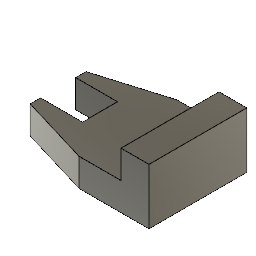
new (Autodesk Fusion 360 design; units mm, degrees)
Autodesk Fusion 360 part; units mm, degrees
sketch "Sketch1" plane through (0, 0, 0) normal (0, 0, 1) x (1, 0, 0)
  line L0 (97.7238, 100.1373) -> (197.7238, 100.1373)
  line L1 (197.7238, 100.1373) -> (197.7238, 30.1373)
  line L2 (197.7238, 30.1373) -> (97.7238, 30.1373)
  line L3 (97.7238, 30.1373) -> (97.7238, 100.1373)
  dimension "d1" = 70
  dimension "d2" = 100
  constraint horizontal L0
  constraint vertical L1
  constraint horizontal L2
  constraint vertical L3
  measures "d1" distance of L0.start L2.end
  measures "d2" distance of L1.end L2.end
extrude "Extrude1" add sketch "Sketch1" along normal blind 20
sketch "Sketch2" plane through (0, 0, 20) normal (0, 0, 1) x (-1, 0, 0)
  line L0 (-97.7238, -30.1373) -> (-197.7238, -30.1373)
  line L1 (-197.7238, -30.1373) -> (-197.7238, -100.1373)
  line L2 (-197.7238, -100.1373) -> (-97.7238, -100.1373)
  line L3 (-97.7238, -100.1373) -> (-97.7238, -30.1373)
  line L4 (-97.7238, -77.6373) -> (-127.7238, -77.6373)
  line L5 (-127.7238, -77.6373) -> (-127.7238, -52.6373)
  line L6 (-127.7238, -52.6373) -> (-97.7238, -52.6373)
  dimension "d5" = 22.5
  dimension "d6" = 22.5
  dimension "d7" = 25
  dimension "d8" = 30
  dimension "d9" = 25
  constraint coincident L3 L6.end
  constraint perpendicular L4 L5
  measures "d5" distance of L2.end L4.start
  measures "d6" distance of L0.start L6.end
  measures "d7" distance of L4.start L6.end
  measures "d8" distance of L4.start L4.end
  measures "d9" distance of L4.end L5.end
extrude "Extrude2" cut sketch "Sketch2" against normal blind 27.453 contours L3 L4 L5 L6
sketch "Sketch3" plane through (0, 0, 20) normal (0, 0, 1) x (-1, 0, 0)
  line L0 (-127.7238, -52.6373) -> (-97.7238, -52.6373)
  line L1 (-97.7238, -52.6373) -> (-97.7238, -30.1373)
  line L2 (-97.7238, -30.1373) -> (-197.7238, -30.1373)
  line L3 (-197.7238, -30.1373) -> (-197.7238, -100.1373)
  line L4 (-197.7238, -100.1373) -> (-97.7238, -100.1373)
  line L5 (-97.7238, -100.1373) -> (-97.7238, -77.6373)
  line L6 (-97.7238, -77.6373) -> (-127.7238, -77.6373)
  line L7 (-127.7238, -77.6373) -> (-127.7238, -52.6373)
  line L8 (-97.7238, -52.6373) -> (-97.7238, -45.1373)
  line L9 (-97.7238, -77.6373) -> (-97.7238, -85.1373)
  line L10 (-147.7238, -30.1373) -> (-147.7238, -100.1373)
  line L11 (-97.7238, -85.1373) -> (-147.7238, -100.1373)
  line L12 (-97.7238, -45.1373) -> (-147.7238, -30.1373)
  dimension "d12" = 7.5
  dimension "d13" = 7.5
  constraint coincident L0.end L1.start
  constraint perpendicular L0 L8
  constraint coincident L5.end L6.start
  constraint coincident L5 L9.end
  constraint midpoint L4 L10.end
  constraint midpoint L2 L10.start
  measures "d12" distance of L0.end L8.end
  measures "d13" distance of L5.end L9.end
extrude "Extrude3" cut sketch "Sketch3" against normal blind 62.472 contours L1 L2 L12
extrude "Extrude4" cut sketch "Sketch3" against normal blind 73.462 contours L4 L5 L11
sketch "Sketch4" plane through (0, 30.1373, 0) normal (0, -1, 0) x (1, 0, 0)
  line L0 (147.7238, 20) -> (147.7238, 0)
  line L1 (147.7238, 0) -> (197.7238, 0)
  line L2 (197.7238, 0) -> (197.7238, 20)
  line L3 (197.7238, 20) -> (147.7238, 20)
  line L4 (197.7238, 20) -> (197.7238, 40)
  line L5 (197.7238, 40) -> (177.7238, 40)
  line L6 (177.7238, 40) -> (177.7238, 20)
  dimension "d18" = 20
  dimension "d19" = 20
  constraint coincident L2.end L3.start
  constraint perpendicular L3 L4
  constraint perpendicular L4 L5
  constraint coincident L3 L6.end
  constraint perpendicular L3 L6
  measures "d18" distance of L2.end L4.end
  measures "d19" distance of L4.end L5.end
extrude "Extrude5" add sketch "Sketch4" against normal blind 70 contours L3 L4 L5 L6
